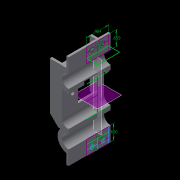
# Autodesk Inventor part: Extruder Holder V2
Saved by Autodesk Inventor 2014 (Build 180170000, 170)
## iProperties
Created: 2015-07-07
Part Number: Extruder Holder V2
Material: Generic
Document SubType Name: Modeling
Designer: Scott
Density: 1 g/cm^3
Appearance: Default
Author: Scott
Autodesk Inventor part; units mm, degrees
ref_plane "YZ Plane" through (0, 0, 0) normal (1, 0, 0) x (0, 1, 0)
ref_plane "XZ Plane" through (0, 0, 0) normal (0, 1, 0) x (-1, 0, 0)
ref_plane "XY Plane" through (0, 0, 0) normal (0, 0, 1) x (1, 0, 0)
ref_plane "Work Plane1" through (0, -60, 0) normal (0, 0, 1) x (-1, 0, 0)
sketch "Sketch1" plane through (0, -60, 0) normal (0, 0, 1) x (-1, 0, 0)
  circle A0 centre (0, 0) radius 4 projected
  circle A1 centre (0, -60) radius 4 projected
  circle A2 centre (0, -60) radius 7.5
  circle A3 centre (0, 0) radius 7.5
  circle A4 centre (0, -60) radius 12.7
  circle A5 centre (0, 0) radius 12.7
  dimension "d0" = 15
  dimension "d1" = 15
  dimension "d2" = 25.4
  dimension "d3" = 25.4
  constraints: 4 centre point, 4 coincident
  measures "d0" diameter of A2
  measures "d1" diameter of A3
  measures "d2" diameter of A4
  measures "d3" diameter of A5
extrude "Extrusion1" add sketch "Sketch1" along normal mid plane 25 contours A4 | A5
sketch "Sketch2" plane through (0, 0, 12.5) normal (0, 0, 1) x (1, 0, 0)
  circle A0 centre (0, 0) radius 12.7 projected
  circle A1 centre (0, -60) radius 7.5 projected
  circle A2 centre (0, -60) radius 12.7 projected
  circle A3 centre (0, 0) radius 7.5 projected
  circle A4 centre (0, 0) radius 12.7 projected
  line L0 (0, -72.7) -> (12.7, -72.7)
  line L1 (12.7, -72.7) -> (12.7, 12.706)
  line L2 (12.7, 12.706) -> (0, 12.7)
  circle A5 centre (0, -60) radius 12.7 projected
  arc A6 (0, -72.7) -> (12.7, -60) centre (0, -60) ccw
  arc A7 (12.7, 0) -> (0, 12.7) centre (0, 0) ccw
  constraints: 6 end point, 6 point on circle, 2 centre point, 2 horizontal, 2 point on line, 2 vertical alignment, 1 horizontal alignment, 1 perpendicular, 3 other
extrude "Extrusion2" add sketch "Sketch2" against normal blind 25 contours A0 L2 L1 | L1 L0 A2
sketch "Sketch3" plane through (12.7, 12.706, 12.5) normal (-0.0004741, 0.9999999, 0) x (0.9999999, 0.0004741, 0)
  line L0 (0, 0) -> (-12.7, 0) projected
  line L1 (0, 0) -> (0, 25) projected
  line L2 (-12.7, 25) -> (0, 25) projected
  line L3 (-12.7, 0) -> (-12.7, 25) projected
  point P0 (-12.706, 12.5)
sketch "Sketch4" plane through (0, -60, -12.5) normal (0, 0, -1) x (-1, 0, 0)
  line L0 (-12.7, 72.706) -> (-12.7, 60) projected
  line L1 (0, 72.7) -> (0, -16.7444)
  line L2 (0, -16.7444) -> (-14.0452, -16.7444)
  line L3 (-14.0452, -16.7444) -> (-14.0452, 76.9468)
  line L4 (-14.0452, 76.9468) -> (0, 72.7)
  constraints: 8 end point, 2 parallel, 1 perpendicular
extrude "Extrusion3" cut sketch "Sketch4" against normal blind 52.3875
sketch "Sketch5" plane through (0, 7.5, -12.5) normal (1, 0, 0) x (0, 0, -1)
  line L0 (-25, 0) -> (-25, 5.2) projected
  line L1 (0, 0) -> (-25, 0) projected
  line L2 (0, 5.2) -> (0, 0) projected
  line L3 (-25, 5.2) -> (0, 5.2) projected
  line L4 (-25, 0) -> (-0.0064, 0)
  line L5 (-0.0064, 0) -> (-0.0064, 16.51)
  line L6 (-0.0064, 16.51) -> (-25, 16.51)
  line L7 (-25, 16.51) -> (-25, 0)
  line L8 (-12.5, 5.2) -> (-12.5032, 16.51)
  line L9 (-12.5016, 10.855) -> (-25, 10.855)
  circle A0 centre (-18.7508, 10.855) radius 2.2225
  line L10 (-0.0064, 10.855) -> (-12.5016, 10.855)
  circle A1 centre (-6.254, 10.855) radius 2.2225
  line L11 (0, -20.2) -> (-25, -20.2) projected
  line L12 (-25, -54.8) -> (0, -54.8) projected
  line L13 (-12.5, -20.2) -> (-12.5, -54.8)
  line L14 (-12.5, -37.5) -> (-25, -37.5)
  line L15 (-25, -75) -> (0, -75) projected
  line L16 (-25, -80.2) -> (-25, -75) projected
  line L17 (-25, -80.2) -> (0, -80.2) projected
  line L18 (0, -75) -> (0, -80.2) projected
  line L19 (-25, -75) -> (0, -75)
  line L20 (0, -75) -> (0, -91.51)
  line L21 (0, -91.51) -> (-25, -91.51)
  line L22 (-25, -91.51) -> (-25, -75)
  line L23 (-12.5, -80.2) -> (-12.5, -91.51)
  line L24 (-25, -85.855) -> (-12.5, -85.855)
  line L25 (-12.5, -85.855) -> (0, -85.855)
  circle A2 centre (-18.75, -85.855) radius 2.2225
  circle A3 centre (-6.25, -85.855) radius 2.2225
  point P0 (-12.5, -7.5)
  dimension "d10" = 24.9936
  dimension "d11" = 16.51
  dimension "d12" = 4.445
  dimension "d13" = 4.445
  dimension "d14" = 16.51
  dimension "d15" = 4.445
  dimension "d16" = 4.445
  constraints: 32 end point, 13 midpoint, 5 perpendicular, 4 centre point, 4 parallel, 4 point on line, 2 horizontal, 1 collinear
  measures "d10" distance of L6.end L5.end
  measures "d11" distance of L5.end L4.end
  measures "d12" diameter of A0
  measures "d13" diameter of A1
  measures "d14" distance of L19.end L20.end
  measures "d15" diameter of A2
  measures "d16" diameter of A3
extrude "Extrusion4" add sketch "Sketch5" against normal blind 2.54
ref_plane "Work Plane2" through (0, -30, -12.5) normal (0, -1, 0) x (1, 0, 0)
sketch "Sketch6" plane through (0, -30, -12.5) normal (0, -1, 0) x (1, 0, 0)
  line L0 (0, 0) -> (0, 25) projected
  line L1 (0, 25) -> (0, 25) projected
  line L2 (0, 25) -> (0, 0) projected
  line L3 (0, 0) -> (0, 0) projected
  line L4 (-7.5, 25) -> (0, 25) projected
  line L5 (0, 0) -> (0, 25) projected
  line L6 (0, 25) -> (0, 25) projected
  line L7 (0, 25) -> (0, 0) projected
  line L8 (0, 0) -> (0, 0) projected
  line L9 (-2.54, 0) -> (-2.54, 25) projected
  line L10 (0, 25) -> (-2.54, 25) projected
  line L11 (0, 25) -> (0, 0) projected
  line L12 (-2.54, 0) -> (0, 0) projected
  line L13 (-7.5, 0) -> (-7.5, 25) projected
  line L14 (-7.5, 0) -> (-10.04, 0)
  line L15 (-10.04, 0) -> (-10.04, 43)
  line L16 (-7.5, 43) -> (-7.5, 0)
  line L17 (-10.04, 0) -> (-21.54, 0)
  line L18 (-21.54, 0) -> (-21.54, -2.54)
  line L19 (-21.54, -2.54) -> (-7.5, -2.54)
  line L20 (-7.5, -2.54) -> (-7.5, 0)
  line L21 (-10.04, 43) -> (-21.54, 43)
  line L22 (-21.54, 43) -> (-21.54, 45.54)
  line L23 (-21.54, 45.54) -> (-7.5, 45.54)
  line L24 (-7.5, 45.54) -> (-7.5, 43)
  point P0 (0, 12.5)
  dimension "d21" = 2.54
  dimension "d22" = 43
  dimension "d23" = 11.5
  dimension "d24" = 2.54
  dimension "d25" = 11.5
  dimension "d26" = 2.54
  constraints: 22 end point, 7 perpendicular, 3 parallel, 1 collinear
  measures "d21" distance of L13.start L14.end
  measures "d22" distance of L14.end L15.end
  measures "d23" distance of L14.end L17.end
  measures "d24" distance of L17.end L18.end
  measures "d25" distance of L15.end L21.end
  measures "d26" distance of L21.end L22.end
extrude "Extrusion6" add sketch "Sketch6" along normal blind 21.59 and the other way blind 42.2275 contours L14 L15 L21 L22 L23 L24 L16 L13 | L20 L19 L18 L17 L14
sketch "Sketch7" plane through (0, -51.59, -12.5) normal (0, -1, 0) x (1, 0, 0)
  line L0 (-10.04, 43) -> (-21.54, 43)
  line L1 (-21.54, 43) -> (-21.54, 0)
  line L2 (-21.54, 0) -> (-10.04, 0)
  line L3 (-10.04, 0) -> (-10.04, 43)
  point P0 (0, 12.5)
  constraints: 8 end point, 2 parallel, 1 horizontal, 1 perpendicular
extrude "Extrusion7" cut sketch "Sketch7" along normal mid plane 152.4
sketch "Sketch8" plane through (0, -60, 12.5) normal (0, 0, 1) x (1, 0, 0)
  line L0 (-7.5, 8.41) -> (-9.5164, 8.41) projected
  arc A0 (-9.5164, 8.41) -> (-2.54, -12.4434) centre (0, 0) ccw projected
  line L1 (-2.54, -24.01) -> (-2.54, -12.4434) projected
  line L2 (0, -24.01) -> (-2.54, -24.01) projected
  line L3 (0, -24.01) -> (0, -7.5) projected
  arc A1 (0, 7.5) -> (0, -7.5) centre (0, 0) ccw projected
  line L4 (0, 7.5) -> (0, 12.7) projected
  arc A2 (0, 12.7) -> (-7.5, 10.2489) centre (0, 0) ccw projected
  line L5 (-7.5, 10.2489) -> (-7.5, 8.41) projected
  line L6 (-7.5, 70.2489) -> (-7.5, 60) projected
  arc A3 (0, 67.5) -> (-7.5, 60) centre (0, 60) ccw projected
  line L7 (0, 84.01) -> (0, 67.5) projected
  line L8 (0, 84.01) -> (-2.54, 84.01) projected
  line L9 (-2.54, 72.4434) -> (-2.54, 84.01) projected
  arc A4 (-2.54, 72.4434) -> (-7.5, 70.2489) centre (0, 60) ccw projected
  line L10 (-7.5, 60) -> (-7.5, 49.7511) projected
  arc A5 (-7.5, 49.7511) -> (0, 47.3) centre (0, 60) ccw projected
  line L11 (0, 47.3) -> (0, 52.5) projected
  arc A6 (-7.5, 60) -> (0, 52.5) centre (0, 60) ccw projected
extrude "Extrusion8" add sketch "Sketch8" along normal up to surface (20.54 mm away)
sketch "Sketch9" plane through (0, -60, -12.5) normal (0, 0, -1) x (-1, 0, 0)
  line L0 (9.5164, 8.41) -> (7.5, 8.41) projected
  line L1 (7.5, 8.41) -> (7.5, 10.2489) projected
  arc A0 (7.5, 10.2489) -> (0, 12.7) centre (0, 0) ccw projected
  line L2 (0, 12.7) -> (0, 7.5) projected
  arc A1 (0, -7.5) -> (0, 7.5) centre (0, 0) ccw projected
  line L3 (0, -24.01) -> (0, -7.5) projected
  line L4 (0, -24.01) -> (2.54, -24.01) projected
  line L5 (2.54, -12.4434) -> (2.54, -24.01) projected
  arc A2 (2.54, -12.4434) -> (9.5164, 8.41) centre (0, 0) ccw projected
  arc A3 (8.3332, 63.0967) -> (2.2038, 68.6125) centre (0, 60) ccw projected
  line L6 (7.5, 60) -> (7.5, 70.2489) projected
  arc A4 (7.5, 70.2489) -> (2.54, 72.4434) centre (0, 60) ccw projected
  line L7 (2.54, 72.7) -> (2.54, 72.4434) projected
  line L8 (0, 72.7) -> (2.54, 72.7) projected
  line L9 (0, 72.7) -> (0, 67.5) projected
  arc A5 (7.5, 60) -> (0, 67.5) centre (0, 60) ccw projected
  line L10 (2.54, 72.7) -> (0, 72.7) projected
  line L11 (2.54, 84.01) -> (2.54, 72.7) projected
  line L12 (0, 84.01) -> (2.54, 84.01) projected
  line L13 (0, 72.7) -> (0, 84.01) projected
  line L14 (7.5, 49.7511) -> (7.5, 60) projected
  arc A6 (0, 52.5) -> (7.5, 60) centre (0, 60) ccw projected
  line L15 (0, 52.5) -> (0, 47.3) projected
  arc A7 (0, 47.3) -> (7.5, 49.7511) centre (0, 60) ccw projected
extrude "Extrusion9" add sketch "Sketch9" along normal up to surface (2.54 mm away)
sketch "Sketch10" plane through (-10.04, -51.59, -12.5) normal (-1, 0, 0) x (0, 0, 1)
  line L0 (43, 0) -> (33.221, 0)
  line L1 (33.221, 0) -> (33.221, 29.845)
  line L2 (33.221, 29.845) -> (43, 29.845)
  line L3 (43, 29.845) -> (43, 0)
  circle A0 centre (33.221, 29.845) radius 1.905
  line L4 (31.316, 29.845) -> (27.506, 29.845)
  line L5 (27.506, 29.845) -> (27.506, 42.545)
  line L6 (27.506, 42.545) -> (27.506, 17.145)
  line L7 (27.506, 17.145) -> (3.376, 17.145)
  line L8 (3.376, 17.145) -> (3.376, 42.545)
  line L9 (3.376, 42.545) -> (27.506, 42.545)
  point P0 (12.5, 51.59)
  dimension "d39" = 3.81
  dimension "d37" = 9.779
  dimension "d38" = 29.845
  dimension "d40" = 3.81
  dimension "d41" = 12.7
  dimension "d42" = 25.4
  dimension "d43" = 24.13
  constraints: 20 end point, 4 parallel, 4 perpendicular, 1 coincident, 1 collinear, 1 horizontal, 1 horizontal alignment, 2 other
  measures "d37" distance of L1.end L2.end
  measures "d38" distance of L0.end L1.end
  measures "d40" distance of L4.start L4.end
  measures "d41" distance of L4.end L5.end
  measures "d42" distance of L5.end L6.end
  measures "d43" distance of L6.end L7.end
extrude "Extrusion10" cut sketch "Sketch10" against normal blind 75.565 contours A0 L2 L1 | L1 L2 A0 | L6 L7 L8 L9 L5
sketch "Sketch11" plane through (-7.5, 12.2275, -15.04) normal (0, 0, -1) x (-1, 0, 0)
  arc A0 (-4.96, -84.6709) -> (2.0164, -63.8175) centre (-7.5, -72.2275) ccw projected
  line L0 (14.04, -63.8175) -> (2.0164, -63.8175) projected
  line L1 (-7.5, -24.9275) -> (-7.5, -21.2725) projected
  arc A1 (-7.5, -24.9275) -> (0, -22.4764) centre (-7.5, -12.2275) ccw projected
  line L2 (0, -46.6725) -> (0, -22.4764) projected
  line L3 (2.54, -46.6725) -> (0, -46.6725) projected
  line L4 (2.54, -21.2725) -> (2.54, -46.6725) projected
  line L5 (2.54, -21.2725) -> (-7.5, -21.2725) projected
  line L6 (2.54, 0) -> (2.54, -63.8175) projected
  line L7 (14.04, -63.8175) -> (2.54, -63.8175) projected
  line L8 (14.04, 0) -> (14.04, -63.8175) projected
  line L9 (2.54, 0) -> (14.04, 0) projected
  line L10 (2.54, -63.8175) -> (2.54, -64.4501)
  line L11 (2.54, -63.8175) -> (2.0164, -63.8175)
  line L12 (2.0164, -63.8175) -> (2.54, -64.4501)
  constraints: 6 end point, 1 collinear, 1 perpendicular, 1 point on circle
extrude "Extrusion11" add sketch "Sketch11" against normal up to surface (48.08 mm away) contours A0 L0 L10
fillet "Fillet1" radius 6.35 2 edges at (-7.5, -49.7511, -13.77) (-7.5, -49.7511, 10.27)
fillet "Fillet2" radius 6.35 2 edges at (-7.5, 10.2489, 10.27) (-7.5, 10.2489, -13.77)
chamfer "Chamfer1" distance 9.525 angle 45 2 edges at (-21.54, -51.59, -13.77) (-21.54, -51.59, 31.77)
body "Solid1"
